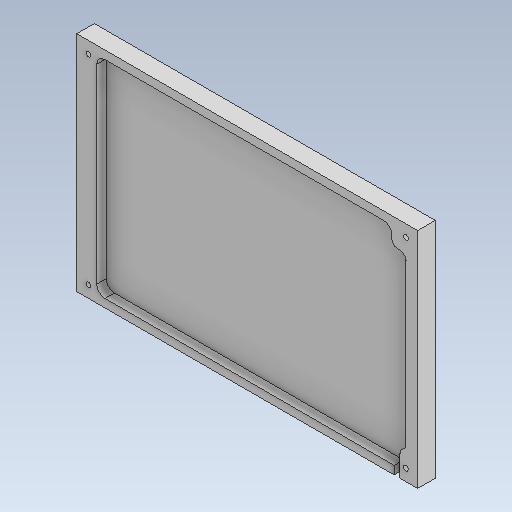
# Autodesk Inventor part: iPadHolder
Saved by Autodesk Inventor 2021.3 (Build 253353000, 353)
## iProperties
Created: 2020-11-06
Part Number: iPadHolder
Material: 一般
Document SubType Name: Modeling
Designer: gisen
Density: 1 g/cm^3
Appearance: 既定
Author: gisen
Autodesk Inventor part; units mm, degrees
ref_plane "YZ Plane" through (0, 0, 0) normal (1, 0, 0) x (0, 1, 0)
sketch "スケッチ1" plane through (0, 0, 0) normal (0, 0, 1) x (1, 0, 0)
  line L0 (-116.8004, 49.1733) -> (173.1996, 49.1733)
  line L1 (173.1996, 49.1733) -> (173.1996, -140.8267)
  line L2 (173.1996, -140.8267) -> (-116.8004, -140.8267)
  line L3 (-116.8004, -140.8267) -> (-116.8004, 49.1733)
  point P0 (0, 0)
  dimension "d0" = 290
  dimension "d1" = 190
  constraints: 8 end point, 2 parallel, 1 horizontal, 1 perpendicular
  measures "d0" distance of L0.start L0.end
  measures "d1" distance of L0.end L1.end
extrude "押し出し1" add sketch "スケッチ1" along normal blind 15
sketch "スケッチ2" plane through (0, 0, 15) normal (0, 0, 1) x (1, 0, 0)
  line L0 (-111.8004, 42.1733) -> (163.1996, 42.1733)
  line L1 (163.1996, 42.1733) -> (163.1996, -133.8267)
  line L2 (163.1996, -133.8267) -> (-111.8004, -133.8267)
  line L3 (-111.8004, -133.8267) -> (-111.8004, 42.1733)
  line L4 (-111.8004, 27.1733) -> (-99.8004, 27.1733)
  line L5 (-99.8004, 27.1733) -> (-99.8004, 42.1733)
  line L6 (-116.8004, 49.1733) -> (-116.8004, -140.8267) projected
  line L7 (-116.8004, -140.8267) -> (173.1996, -140.8267) projected
  line L8 (173.1996, 49.1733) -> (-116.8004, 49.1733) projected
  line L9 (28.1996, -45.8267) -> (-116.8004, -45.8267)
  line L10 (28.1996, -45.8267) -> (28.1996, 49.1733)
  line L11 (168.1996, 27.1733) -> (158.1996, 27.1733)
  line L12 (158.1996, 27.1733) -> (158.1996, 42.1733)
  line L13 (-111.8004, -118.8267) -> (-99.8004, -118.8267)
  line L14 (-99.8004, -118.8267) -> (-99.8004, -133.8267)
  line L15 (158.1996, -118.8267) -> (158.1996, -133.8267)
  line L16 (168.1996, -118.8267) -> (158.1996, -118.8267)
  line L17 (-99.8004, 27.1733) -> (-99.8004, -118.8267)
  line L18 (158.1996, 27.1733) -> (151.1996, 27.1733)
  line L19 (151.1996, 27.1733) -> (151.1996, 42.1733)
  line L20 (158.1996, -118.8267) -> (151.1996, -118.8267)
  line L21 (151.1996, -118.8267) -> (151.1996, -133.8267)
  point P0 (0, 0)
  point P1 (163.1996, -118.8267)
  point P2 (163.1996, 27.1733)
  point P3 (158.1996, 42.1733)
  point P4 (-111.8004, -118.8267)
  point P5 (158.1996, -133.8267)
  dimension "d4" = 15
  dimension "d5" = 275
  dimension "d6" = 5
  dimension "d7" = 7
  dimension "d8" = 7
  dimension "d9" = 12
  dimension "d15" = 7
  constraints: 38 end point, 6 point on line, 4 perpendicular, 4 symmetric about line, 3 horizontal, 2 midpoint, 2 parallel, 1 vertical
  measures "d4" distance of L4.end L5.end
  measures "d5" distance of L0.start L0.end
  measures "d6" distance between parallel lines of L6 L3
  measures "d7" distance between parallel lines of L7 L2
  measures "d8" distance between parallel lines of L8 L0
  measures "d9" distance of L4.start L4.end
  measures "d15" distance of L12.start L18.end
ref_plane "作業平面1" through (28.1996, -140.8267, 0) normal (-1, 0, 0) x (0, 0, 1)
ref_plane "作業平面2" through (-116.8004, -45.8267, 0) normal (0, 1, 0) x (1, 0, 0)
extrude "押し出し2" cut sketch "スケッチ2" against normal blind 8 contours L0 L10 L9 L17 L5 | L0 L19 L18 L11 L1 L16 L20 L21 L2 L14 L17 L9 L10 | L21 L20 L15 L2
sketch "スケッチ3" plane through (-116.8004, -140.8267, 0) normal (0, -1, 0) x (1, 0, 0)
  line L0 (275, 15) -> (275, 7) projected
  line L1 (275, 7) -> (17, 7) projected
  line L2 (275, 7) -> (270, 7)
  line L3 (270, 7) -> (270, 15)
  line L4 (0, 15) -> (290, 15) projected
  line L5 (270, 7) -> (270, 0)
  line L6 (290, 0) -> (0, 0) projected
  line L7 (275, 15) -> (275, 7) projected
  line L8 (275, 0) -> (275, 7)
  point P0 (116.8004, 0)
  dimension "d12" = 5
  constraints: 8 end point, 4 point on line, 1 collinear, 1 perpendicular, 1 vertical
  measures "d12" distance of L2.end L0.end
extrude "押し出し3" cut sketch "スケッチ3" against normal blind 7
sketch "スケッチ4" plane through (0, 0, 15) normal (0, 0, 1) x (1, 0, 0)
  circle A0 centre (-106.8004, 39.1733) radius 2.25 projected
  circle A1 centre (163.1996, 39.1733) radius 2.25 projected
  circle A2 centre (163.1996, -130.8267) radius 2.25 projected
  line L0 (153.1996, -133.8267) -> (-99.8004, -133.8267) projected
  line L1 (-99.8004, -133.8267) -> (-99.8004, 42.1733) projected
  line L2 (-99.8004, 42.1733) -> (151.1996, 42.1733) projected
  line L3 (151.1996, 42.1733) -> (151.1996, 27.1733) projected
  line L4 (151.1996, 27.1733) -> (163.1996, 27.1733) projected
  line L5 (163.1996, 27.1733) -> (163.1996, -118.8267) projected
  line L6 (163.1996, -118.8267) -> (158.1996, -118.8267) projected
  line L7 (158.1996, -118.8267) -> (158.1996, -140.8267) projected
  line L8 (-116.8004, -140.8267) -> (153.1996, -140.8267) projected
  line L9 (173.1996, -140.8267) -> (173.1996, 49.1733) projected
  line L10 (173.1996, 49.1733) -> (-116.8004, 49.1733) projected
  line L11 (-116.8004, 49.1733) -> (-116.8004, -140.8267) projected
  line L12 (158.1996, -140.8267) -> (173.1996, -140.8267) projected
  circle A3 centre (-106.8004, -130.8267) radius 2.25 projected
  line L13 (153.1996, -140.8267) -> (153.1996, -133.8267) projected
  point P0 (0, 0)
hole "穴1" at (-106.8004, 39.1733, 15) at (-106.8004, -130.8267, 15) at (163.1996, -130.8267, 15) at (163.1996, 39.1733, 15) direction (0, 0, -1) diameter 4.2 depth 4
fillet "フィレット2" radius 7 3 edges at (-99.8004, 42.1733, 11) (-99.8004, -133.8267, 11) (151.1996, 42.1733, 11)
fillet "フィレット3" radius 5 4 edges at (151.1996, 27.1733, 11) (163.1996, 27.1733, 11) (158.1996, -118.8267, 11) (163.1996, -118.8267, 11)
sketch "スケッチ5" plane through (0, 0, 0) normal (0, 0, -1) x (-1, 0, 0)
  line L0 (-143.1996, 41.1733) -> (92.8004, 41.1733) projected
  line L1 (92.8004, -133.8267) -> (-143.1996, -133.8267) projected
  line L2 (99.8004, 34.1733) -> (99.8004, -126.8267) projected
  line L3 (-163.1996, 22.1733) -> (-163.1996, -113.8267) projected
  line L4 (-173.1996, -140.8267) -> (-173.1996, 49.1733) projected
  line L5 (-28.1996, 87.1733) -> (-28.1996, -178.8267) projected
  line L6 (-231.1996, -45.8267) -> (174.8004, -45.8267) projected
  line L7 (-173.1996, 49.1733) -> (116.8004, 49.1733) projected
  point P0 (0, 0)
  point P1 (-98.1996, 41.6733)
  point P2 (41.8004, 41.6733)
  point P3 (-98.1996, -133.3267)
  point P4 (41.8004, -133.3267)
  point P5 (-165.6996, -30.8267)
  point P6 (-165.6996, -60.8267)
  point P7 (109.3004, -30.8267)
  point P8 (109.3004, -60.8267)
  point P9 (-68.1996, 41.6733)
  point P10 (11.8004, 41.6733)
  point P11 (-68.1996, -133.3267)
  point P12 (11.8004, -133.3267)
  dimension "d26" = 75
  dimension "d27" = 7.5
  dimension "d28" = 15
  dimension "d29" = 7.5
  dimension "d30" = 30
  dimension "d31" = 7.5
  constraints: 9 symmetric about line
  measures "d26" distance from line of L4 point (-98.2, 41.673)
  measures "d27" distance from line of L7 point (-98.2, 41.673)
  measures "d28" distance from line of L6 point (-165.7, -30.827)
  measures "d29" distance from line of L4 point (-165.7, -30.827)
  measures "d30" distance of point (-68.2, 41.673) point (-98.2, 41.673)
  measures "d31" distance from line of L7 point (-68.2, 41.673)
hole "穴2" at (98.1996, 41.6733, 0) at (-41.8004, 41.6733, 0) at (98.1996, -133.3267, 0) at (-41.8004, -133.3267, 0) at (165.6996, -30.8267, 0) at (165.6996, -60.8267, 0) at (-109.3004, -30.8267, 0) at (-109.3004, -60.8267, 0) at (68.1996, 41.6733, 0) at (-11.8004, 41.6733, 0) at (68.1996, -133.3267, 0) at (-11.8004, -133.3267, 0) direction (0, 0, 1) diameter 4.2 depth 4
